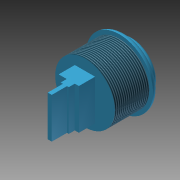
# Autodesk Inventor part: OBSN-30-B
Saved by Autodesk Inventor 2013 (Build 170138000, 138)
## iProperties
Created: 2012-06-18
Part Number: OBSN-30-B
Material: Nylon 6
Document SubType Name: Modeling
Designer: xylzlyx
Density: 1 g/cm^3
Author: xylzlyx
Autodesk Inventor part; units mm, degrees
ref_plane "YZ Plane" through (0, 0, 0) normal (1, 0, 0) x (0, 1, 0)
ref_plane "XZ Plane" through (0, 0, 0) normal (0, 1, 0) x (-1, 0, 0)
ref_plane "XY Plane" through (0, 0, 0) normal (0, 0, 1) x (1, 0, 0)
sketch "Sketch1" plane through (0, 0, 0) normal (0, 1, 0) x (-1, 0, 0)
  circle A0 centre (0, 0) radius 12.5
  circle A1 centre (0, 0) radius 16.6
  circle A2 centre (0, 0) radius 18
  circle A3 centre (0, 0) radius 14.75
  dimension "d0" = 25
  dimension "d1" = 33.2
  dimension "d2" = 36
  dimension "d3" = 29.5
  constraints: 4 centre point, 4 coincident
  measures "d0" diameter of A0
  measures "d1" diameter of A1
  measures "d2" diameter of A2
  measures "d3" diameter of A3
extrude "Extrusion1" add sketch "Sketch1" along normal blind 3 contours A1 | A3
sketch "Sketch2" plane through (0, 0, 0) normal (0, -1, 0) x (1, 0, 0)
  circle A0 centre (0, 0) radius 12.5 projected
  circle A1 centre (0, 0) radius 12.5
  circle A2 centre (0, 0) radius 16.6
  circle A3 centre (0, 0) radius 18
  circle A4 centre (0, 0) radius 14.75
  dimension "d6" = 25
  dimension "d7" = 33.2
  dimension "d8" = 36
  dimension "d9" = 29.5
  constraints: 4 centre point, 4 coincident
  measures "d6" diameter of A1
  measures "d7" diameter of A2
  measures "d8" diameter of A3
  measures "d9" diameter of A4
extrude "Extrusion2" add sketch "Sketch2" against normal blind 6.4 contours A0
fillet "Fillet1" radius 1.5 1 edges at (-12.5, 6.4, 0)
fillet "Fillet2" radius 2.95 1 edges at (16.6, 3, 0)
sketch "Sketch5" plane through (0, 0, 0) normal (0, -1, 0) x (1, 0, 0)
  circle A0 centre (0, 0) radius 16.6 projected
  circle A1 centre (0, 0) radius 14.75
  dimension "d23" = 29.5
  constraints: 1 centre point, 1 coincident
  measures "d23" diameter of A1
extrude "Extrusion5" add sketch "Sketch5" along normal blind 17 contours A1
sketch "Sketch7" plane through (0, -17, 0) normal (0, -1, 0) x (1, 0, 0)
  line L0 (4.9559, 9.4025) -> (-5.0441, 9.4025)
  line L1 (-5.0441, 9.4025) -> (-5.0441, -10.5975)
  line L2 (-5.0441, -10.5975) -> (4.9559, -10.5975)
  line L3 (4.9559, -10.5975) -> (4.9559, 9.4025)
  point P0 (0, 0)
  dimension "d30" = 10
  dimension "d32" = 20
  constraints: 8 end point, 2 parallel, 1 horizontal, 1 perpendicular
  measures "d30" distance of L0.start L0.end
  measures "d32" distance of L2.end L0.start
extrude "Extrusion7" add sketch "Sketch7" along normal blind 8
sketch "Sketch8" plane through (0, -25, 0) normal (0, -1, 0) x (1, 0, 0)
  line L0 (-1.0467, 9.4141) -> (2.9533, 9.4141)
  line L1 (2.9533, 9.4141) -> (2.9533, -10.5859)
  line L2 (2.9533, -10.5859) -> (-1.0467, -10.5859)
  line L3 (-1.0467, -10.5859) -> (-1.0467, 9.4141)
  point P0 (0, 0)
  dimension "d35" = 4
  dimension "d37" = 20
  constraints: 8 end point, 2 parallel, 1 horizontal, 1 perpendicular
  measures "d35" distance of L0.start L0.end
  measures "d37" distance of L0.end L1.end
extrude "Extrusion8" add sketch "Sketch8" along normal blind 3
thread "Thread1" size "M30x1" class "6g" standard "ANSI Metric M Profile" full length
sketch "Sketch10" plane through (0, -28, 0) normal (0, -1, 0) x (1, 0, 0)
  line L0 (0.0695, 9.4148) -> (2.0695, 9.4148)
  line L1 (2.0695, 9.4148) -> (2.0695, -10.5852)
  line L2 (2.0695, -10.5852) -> (0.0695, -10.5852)
  line L3 (0.0695, -10.5852) -> (0.0695, 9.4148)
  point P0 (0, 0)
  dimension "d46" = 20
  dimension "d48" = 2
  constraints: 8 end point, 2 parallel, 1 horizontal, 1 perpendicular
  measures "d46" distance of L0.end L1.end
  measures "d48" distance of L1.end L2.end
extrude "Extrusion10" add sketch "Sketch10" along normal blind 7.5
body "Solid1"
